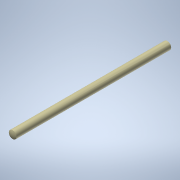
# Autodesk Inventor part: Centre Pin
Saved by Autodesk Inventor 2020.2 (Build 242310000, 310)
## iProperties
Created: 2013-11-30
Part Number: Centre Pin
Material: Generic
Document SubType Name: Modeling
Designer: NiveshandNisheeth
Density: 1 g/cm^3
Appearance: Nylon 6
Author: NiveshandNisheeth
Autodesk Inventor part; units mm, degrees
ref_plane "YZ Plane" through (0, 0, 0) normal (1, 0, 0) x (0, 1, 0)
sketch "Sketch1" plane through (0, 0, 0) normal (0, 0, 1) x (1, 0, 0)
  circle A0 centre (0, 4.7625) radius 3.175 projected
  point P0 (0, 0)
ref_plane "Work Plane1" through (-31.75, 0, 63.5) normal (0, 0, 1) x (1, 0, 0)
ref_plane "Work Plane2" through (-31.75, 0, -63.5) normal (0, 0, -1) x (0, 1, 0)
extrude "Extrusion1" add sketch "Sketch1" against normal up to surface (127 mm away) from surface at 63.5
sketch "Sketch2" plane through (0, 0, 0) normal (1, 0, 0) x (0, 1, 0)
  line L0 (1.5875, 63.5) -> (7.9375, 63.5) projected
  line L1 (4.7625, 63.5) -> (7.9375, 63.5)
  line L2 (7.9375, 63.5) -> (7.9375, 64.2937)
  line L3 (7.9375, 64.2937) -> (4.7625, 64.2937)
  line L4 (4.7625, 64.2937) -> (4.7625, 63.5)
  arc A0 (7.9375, 63.5) -> (4.7625, 64.2937) centre (4.7625, 57.5469) ccw
  point P0 (0, 0)
  dimension "d2" = 0.7937
  constraints: 8 end point, 2 parallel, 2 point on circle, 1 centre point, 1 collinear, 1 midpoint, 1 perpendicular, 1 tangent
  measures "d2" distance between parallel lines of L1 L3
revolve "Revolution1" add sketch "Sketch2" angle 360 about axis through (0, 4.7625, 64.2937) along (0, 0, -1) contours L4 A0 L0
mirror "Mirror1" about plane through (0, 0, 0) normal (0, 0, 1) of "Revolution1"
body "Solid1"
